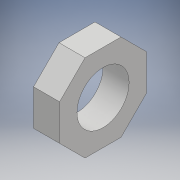
# Autodesk Inventor part: Nuy
Saved by Autodesk Inventor 2018 (Build 220112000, 112)
## iProperties
Created: 2019-05-13
Part Number: Nuy
Material: Generic
Document SubType Name: Modeling
Designer: aal_9
Density: 1 g/cm^3
Appearance: Default
Author: aal_9
Autodesk Inventor part; units mm, degrees
ref_plane "YZ Plane" through (0, 0, 0) normal (1, 0, 0) x (0, 1, 0)
ref_plane "XZ Plane" through (0, 0, 0) normal (0, 1, 0) x (-1, 0, 0)
ref_plane "XY Plane" through (0, 0, 0) normal (0, 0, 1) x (1, 0, 0)
sketch "Sketch1" plane through (0, 0, 0) normal (1, 0, 0) x (0, 1, 0)
  line L0 (-2.0698, 5.0005) -> (2.0723, 4.9995)
  line L1 (2.0723, 4.9995) -> (5.0005, 2.0698)
  line L2 (5.0005, 2.0698) -> (4.9995, -2.0723)
  line L3 (4.9995, -2.0723) -> (2.0698, -5.0005)
  line L4 (2.0698, -5.0005) -> (-2.0723, -4.9995)
  line L5 (-2.0723, -4.9995) -> (-5.0005, -2.0698)
  line L6 (-5.0005, -2.0698) -> (-4.9995, 2.0723)
  line L7 (-4.9995, 2.0723) -> (-2.0698, 5.0005)
  circle A0 centre (0, 0) radius 3
  dimension "d0" = 5
  dimension "d1" = 6
  constraints: 16 end point, 2 coincident, 1 centre point, 17 other
  measures "d0" distance from line of L2 point (0, 0)
  measures "d1" diameter of A0
extrude "Extrusion1" add sketch "Sketch1" along normal blind 3
body "Solid1"
